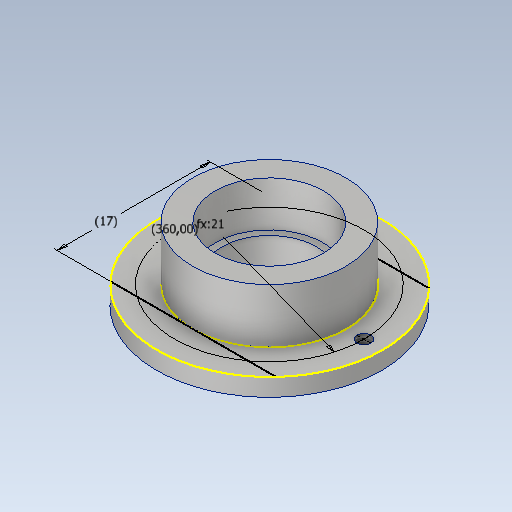
# Autodesk Inventor part: LowerArm_JointFixation
Saved by Autodesk Inventor 2021.4 (Build 254397000, 397)
## iProperties
Created: 2022-07-05
Part Number: LowerArm_JointFixation
Material: Aluminum 6061
Document SubType Name: Modeling
Designer: alexw
Density: 2.7 g/cm^3
Appearance: Aluminum - Flat
Mass: 2.82163 g
Surface Area: 12.908 cm^2
Volume: 1.04505 cm^3
JointFixation_DiaOut: 25,000 mm
JointFixation_FixHole_Dia: 21,000 mm
Bearing_OuterRing_Dia: 10,500 mm
ShaftFixation_UpperLower_Height: 8,000 mm
LowerArm_BearingFixFlansch_Width: 17,000 mm
Author: alexw
Autodesk Inventor part; units mm, degrees
ref_plane "YZ Plane" through (0, 0, 0) normal (1, 0, 0) x (0, 1, 0)
ref_plane "XZ Plane" through (0, 0, 0) normal (0, 1, 0) x (-1, 0, 0)
ref_plane "XY Plane" through (0, 0, 0) normal (0, 0, 1) x (1, 0, 0)
sketch "Sketch1" plane through (0, 0, 0) normal (0, 0, 1) x (1, 0, 0)
  line L0 (0, 0) -> (0, 8) construction
  line L1 (6, 0) -> (12.5, 0)
  line L2 (12.5, 0) -> (12.5, 2)
  line L3 (12.5, 2) -> (8.5, 2)
  line L4 (8.5, 2) -> (8.5, 8)
  line L5 (8.5, 8) -> (6, 8)
  line L6 (6, 8) -> (6, 3)
  line L7 (6, 3) -> (5.25, 3)
  line L8 (5.25, 3) -> (5.25, 0)
  line L9 (5.25, 0) -> (6, 0)
  line L10 (6, 0) -> (6, 0)
  line L11 (10.5, 2) -> (10.5, 0) construction
  line L12 (9.5, 2) -> (11.5, 2) construction
  line L13 (11.5, 2) -> (11.5, 0) construction
  line L14 (11.5, 0) -> (9.5, 0) construction
  line L15 (9.5, 0) -> (9.5, 2) construction
  line L16 (9.5, 2) -> (11.5, 0) construction
  line L17 (11.5, 2) -> (9.5, 0) construction
  line L18 (-2.5, 0) -> (15, 0) construction
  point P0 (10.5, 1)
  dimension "d1" = 2
  dimension "d3" = 2
  dimension "d4" = 12
  dimension "d5" = 2.5
  dimension "JointFixation_FixHole_Dia" = 21
  dimension "ShaftFixation_UpperLower_Height" = 8
  dimension "Bearing_OuterRing_Dia" = 10.5
  dimension "JointFixation_DiaOut" = 25
  dimension "d28" = 5
  constraints: 36 end point, 10 perpendicular, 4 midpoint, 3 collinear, 3 point on line, 2 horizontal, 2 parallel, 1 vertical
  measures "d1" distance between parallel lines of L13 L15
  measures "d3" distance between parallel lines of L18 L3
  measures "d4" diameter of L10 L0
  measures "d5" distance between parallel lines of L4 L6
  measures "JointFixation_FixHole_Dia" diameter of L11 L0
  measures "ShaftFixation_UpperLower_Height" distance between parallel lines of L1 L5
  measures "Bearing_OuterRing_Dia" diameter of L8 L0
  measures "JointFixation_DiaOut" diameter of L2 L0
  measures "d28" distance between parallel lines of L7 L5
revolve "Revolution1" add sketch "Sketch1" angle 360 about axis through (0, 0, 0) along (0, 1, 0)
sketch "Sketch2" plane through (0, 2, 0) normal (0, 1, 0) x (1, 0, 0)
  circle A0 centre (0, 0) radius 8.5 projected
  circle A1 centre (0, 0) radius 12.5 projected
  line L0 (-9.1652, 8.5) -> (9.1652, 8.5)
  line L1 (-9.1652, -8.5) -> (9.1652, -8.5)
  circle A2 centre (0, 0) radius 10.5 construction
  line L2 (0, 0) -> (-10.5, 0) construction
  point P0 (0, 0)
  point P1 (10.5, 0)
  dimension "d14" = 21
  dimension "d17" = 360
  dimension "LowerArm_BearingFixFlansch_Width" = 17
  constraints: 6 end point, 4 point on circle, 3 horizontal, 2 tangent, 1 coincident, 1 horizontal alignment, 5 other
  measures "LowerArm_BearingFixFlansch_Width" distance between parallel lines of L1 L0
hole "Hole1" at (-10.5, 2, 0) at (10.5, 2, 0) direction (0, -1, 0) diameter 1.567 end through all thread size "M2x0.4" class "6H" standard "ISO Metric profile"
equation "\"d14\" = JointFixation_FixHole_Dia"
body "Solid1"
